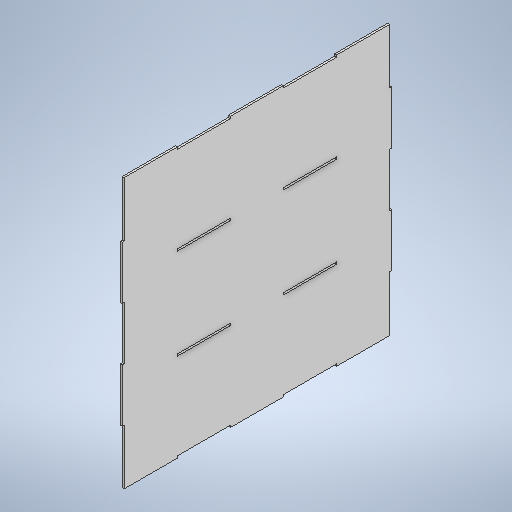
# Autodesk Inventor part: Pared estanteria
Saved by Autodesk Inventor 2025.1 (Build 291241020, 241B)
## iProperties
Created: 2024-11-12
Part Number: Pared estanteria
Material: Generic
Document SubType Name: Modeling
Designer: marco
Density: 1 g/cm^3
Appearance: Default
Author: marco
Autodesk Inventor part; units mm, degrees
ref_plane "YZ Plane" through (0, 0, 0) normal (1, 0, 0) x (0, 1, 0)
ref_plane "XZ Plane" through (0, 0, 0) normal (0, 1, 0) x (-1, 0, 0)
ref_plane "XY Plane" through (0, 0, 0) normal (0, 0, 1) x (1, 0, 0)
sketch "Sketch1" plane through (0, 0, 0) normal (1, 0, 0) x (0, 1, 0)
  line L0 (0, 0) -> (400, 0)
  line L1 (400, 0) -> (400, -400)
  line L2 (400, -400) -> (0, -400)
  line L3 (0, -400) -> (0, 0)
  line L4 (400, 0) -> (403, 0)
  line L5 (403, 0) -> (403, -80)
  line L6 (403, -80) -> (400, -80)
  line L7 (400, -400) -> (403, -400)
  line L8 (403, -400) -> (403, -320)
  line L9 (403, -320) -> (400, -320)
  line L10 (400, -160) -> (403, -160)
  line L11 (403, -160) -> (403, -240)
  line L12 (403, -240) -> (400, -240)
  line L13 (80, 0) -> (80, 3)
  line L14 (80, 3) -> (160, 3)
  line L15 (160, 3) -> (160, 0)
  line L16 (320, 0) -> (320, 3)
  line L17 (320, 3) -> (240, 3)
  line L18 (240, 3) -> (240, 0)
  line L19 (200, 0) -> (200, -400) construction
  line L20 (0, -200) -> (400, -200) construction
  line L21 (0, -400) -> (400, -400)
  line L22 (80, -400) -> (80, -403)
  line L23 (80, -403) -> (160, -403)
  line L24 (160, -403) -> (160, -400)
  line L25 (320, -400) -> (320, -403)
  line L26 (320, -403) -> (240, -403)
  line L27 (240, -403) -> (240, -400)
  line L28 (0, 0) -> (0, -400)
  line L29 (0, 0) -> (-3, 0)
  line L30 (-3, 0) -> (-3, -80)
  line L31 (-3, -80) -> (0, -80)
  line L32 (0, -400) -> (-3, -400)
  line L33 (-3, -400) -> (-3, -320)
  line L34 (-3, -320) -> (0, -320)
  line L35 (0, -160) -> (-3, -160)
  line L36 (-3, -160) -> (-3, -240)
  line L37 (-3, -240) -> (0, -240)
  line L38 (0, 0) -> (130, 0)
  line L39 (130, 0) -> (133, 0)
  line L40 (133, 0) -> (267, 0)
  line L41 (267, 0) -> (270, 0)
  line L42 (133, -80) -> (130, -80)
  line L43 (133, -80) -> (133, -160)
  line L44 (133, -160) -> (130, -160)
  line L45 (130, -320) -> (133, -320)
  line L46 (133, -320) -> (133, -240)
  line L47 (133, -240) -> (130, -240)
  line L48 (133, -80) -> (130, -80)
  line L49 (130, -80) -> (130, -160)
  line L50 (130, -320) -> (130, -240)
  line L51 (400, -200) -> (0, -200) construction
  line L52 (267, -80) -> (270, -80)
  line L53 (267, -80) -> (267, -160)
  line L54 (267, -160) -> (270, -160)
  line L55 (270, -320) -> (267, -320)
  line L56 (267, -320) -> (267, -240)
  line L57 (267, -240) -> (270, -240)
  line L58 (267, -80) -> (270, -80)
  line L59 (270, -80) -> (270, -160)
  line L60 (270, -320) -> (270, -240)
  dimension "d0" = 400
  dimension "d1" = 400
  dimension "d2" = 3
  dimension "d3" = 80
  dimension "d4" = 3
  dimension "d5" = 80
  dimension "d6" = 80
  dimension "d7" = 3
  dimension "d8" = 80
  dimension "d13" = 3
  dimension "d14" = 80
  dimension "d17" = 130
  dimension "d18" = 3
  dimension "d19" = 134
  dimension "d20" = 3
  dimension "d21" = 80
  dimension "d22" = 80
  dimension "d24" = 80
  dimension "d25" = 3
  constraints: 120 end point, 28 symmetric about line, 24 point on line, 5 perpendicular, 5 vertical, 3 horizontal, 3 midpoint, 1 parallel, 12 other
  measures "d0" distance of L1.end L2.end
  measures "d1" distance of L1.start L1.end
  measures "d2" distance of L1.start L4.end
  measures "d3" distance of L4.end L5.end
  measures "d4" distance of L1.end L7.end
  measures "d5" distance of L7.end L8.end
  measures "d6" distance of L6.end L10.start
  measures "d7" distance of L10.start L10.end
  measures "d8" distance of L10.end L11.end
  measures "d13" distance of L16.start L16.end
  measures "d14" distance of L16.end L17.end
  measures "d17" distance of L3.end L38.end
  measures "d18" distance of L38.end L39.end
  measures "d19" distance of L39.end L40.end
  measures "d20" distance of L40.end L41.end
  measures "d21" distance of L39.end L42.start
  measures "d22" distance of L42.start L43.end
  measures "d24" distance of L45.end L46.end
  measures "d25" distance of L42.start L42.end
extrude "Extrusion1" add sketch "Sketch1" along normal blind 3
body "Solid1"
